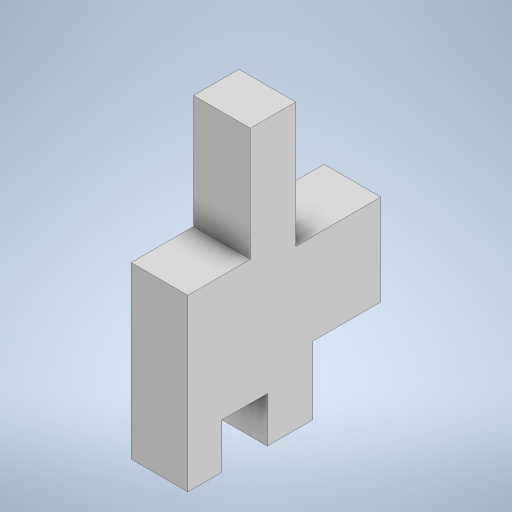
# Autodesk Inventor part: Деталь2
Saved by Autodesk Inventor 2023.2 (Build 272271030, 271C)
## iProperties
Created: 2023-10-26
Part Number: Деталь2
Material: Типовые
Document SubType Name: Sheet Metal
Designer: Elisey
Density: 1 g/cm^3
Sheet Metal Rule: По умолчанию_мм
Appearance: По умолчанию
Author: Elisey
Autodesk Inventor part; units mm, degrees
ref_plane "YZ Plane" through (0, 0, 0) normal (1, 0, 0) x (0, 1, 0)
ref_plane "XZ Plane" through (0, 0, 0) normal (0, 1, 0) x (-1, 0, 0)
ref_plane "XY Plane" through (0, 0, 0) normal (0, 0, 1) x (1, 0, 0)
sketch "Эскиз1" plane through (0, 0, 0) normal (1, 0, 0) x (0, 1, 0)
  line L0 (0.3766, -35.0912) -> (12.3766, -35.0912)
  line L1 (12.3766, -35.0912) -> (12.3766, -47.0912)
  line L2 (12.3766, -47.0912) -> (28.3766, -47.0912)
  line L3 (28.3766, -32.0912) -> (50.3766, -32.0912)
  line L4 (50.3766, -32.0912) -> (50.3766, -24.0912)
  line L5 (50.3766, -24.0912) -> (30.3766, -24.0912)
  line L6 (30.3766, -24.0912) -> (30.3766, -13.0912)
  line L7 (28.3766, -47.0912) -> (28.3766, -32.0912)
  line L8 (0.3766, -35.0912) -> (0.3766, -27.0912)
  line L9 (0.3766, -27.0912) -> (8.3766, -27.0912)
  line L10 (8.3766, -27.0912) -> (8.3766, -19.0912)
  line L11 (8.3766, -19.0912) -> (0.3766, -19.0912)
  line L12 (0.3766, -19.0912) -> (0.3766, -13.0912)
  line L13 (0.3766, -13.0912) -> (30.3766, -13.0912)
  point P0 (0, 0)
  point P1 (-47.0655, -24.8908)
  constraints: 28 end point, 7 perpendicular, 2 point on line
extrude "Выдавливание1" add sketch "Эскиз1" along normal blind 10
equation "\"Радиус_гибки\" = Толщина"
equation "\"Ширина_просечки\" = Толщина"
equation "\"Глубина_просечки\" = 0.5 * Толщина"
equation "\"Размер_просечки\" = 4 * Толщина"
equation "\"Мин_остаток\" = 2 * Толщина"
equation "\"Радиус_перехода\" = Радиус_гибки"
equation "\"Радиус_Якоби\" = Радиус_гибки"
equation "\"Размер_зазора\" = Толщина"
equation "\"Толщина\" = 0.5"
